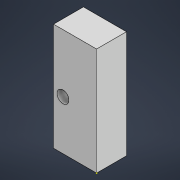
# Autodesk Inventor part: 200515
Saved by Autodesk Inventor 2022.2 (Build 262287000, 287)
## iProperties
Created: 2022-09-12
Part Number: 200515
Material: Generic
Document SubType Name: Modeling
Designer: robotics
Mass: 1.78241 g
Surface Area: 10.6977 cm^2
Volume: 1.78241 cm^3
Density: 1 g/cm^3
Appearance: Default
Author: robotics
Autodesk Inventor part; units mm, degrees
ref_plane "YZ Plane" through (0, 0, 0) normal (1, 0, 0) x (0, 1, 0)
ref_plane "XZ Plane" through (0, 0, 0) normal (0, 1, 0) x (-1, 0, 0)
ref_plane "XY Plane" through (0, 0, 0) normal (0, 0, 1) x (1, 0, 0)
sketch "Sketch1" plane through (0, 0, 0) normal (0, 1, 0) x (-1, 0, 0)
  line L0 (0, 0) -> (10.1736, 0)
  line L1 (10.1736, 0) -> (10.1736, 7.068)
  line L2 (10.1736, 7.068) -> (0, 7.068)
  line L3 (0, 7.068) -> (0, 0)
  constraints: 8 end point, 2 parallel, 1 horizontal, 1 perpendicular
extrude "Extrusion1" add sketch "Sketch1" along normal blind 25.4
sketch "Sketch2" plane through (-10.1736, 0, 7.068) normal (0, 0, 1) x (1, 0, 0)
  point P0 (10.1736, 0)
sketch "Sketch3" plane through (-10.1736, 0, 7.068) normal (0, 0, 1) x (1, 0, 0)
  circle A0 centre (2.2327, 11.6549) radius 1.4082
  point P0 (10.1736, 0)
  constraints: 1 centre point
extrude "Extrusion2" cut sketch "Sketch3" against normal blind 25.4
body "Solid1"
